Autodesk Fusion 360 part; units mm, degrees
(part 23 of 40)
  line L3449 (13.3622, 59.5542) -> (13.369, 59.5843) construction
  line L3450 (13.369, 59.5843) -> (13.3833, 59.6444) construction
  line L3451 (13.3833, 59.6444) -> (13.4071, 59.7338) construction
  line L3452 (13.4071, 59.7338) -> (13.4435, 59.8517) construction
  line L3453 (13.4435, 59.8517) -> (13.4951, 59.9973) construction
  line L3454 (13.4951, 59.9973) -> (13.5511, 60.1416) construction
  line L3455 (13.5511, 60.1416) -> (13.6099, 60.2852) construction
  line L3456 (13.6099, 60.2852) -> (13.6701, 60.4283) construction
  line L3457 (13.6701, 60.4283) -> (13.7313, 60.5711) construction
  line L3458 (13.7313, 60.5711) -> (13.7935, 60.7136) construction
  line L3459 (13.7935, 60.7136) -> (13.8571, 60.8557) construction
  line L3460 (13.8571, 60.8557) -> (13.9226, 60.9971) construction
  line L3461 (13.9226, 60.9971) -> (13.9902, 61.1379) construction
  line L3462 (13.9902, 61.1379) -> (14.06, 61.2779) construction
  line L3463 (14.06, 61.2779) -> (14.1316, 61.4173) construction
  line L3464 (14.1316, 61.4173) -> (14.205, 61.5561) construction
  line L3465 (14.205, 61.5561) -> (14.2797, 61.6944) construction
  line L3466 (14.2797, 61.6944) -> (14.3557, 61.8322) construction
  line L3467 (14.3557, 61.8322) -> (14.4327, 61.9697) construction
  line L3468 (14.4327, 61.9697) -> (14.5109, 62.1067) construction
  line L3469 (14.5109, 62.1067) -> (14.5904, 62.2432) construction
  line L3470 (14.5904, 62.2432) -> (14.6711, 62.3792) construction
  line L3471 (14.6711, 62.3792) -> (14.753, 62.5148) construction
  line L3472 (14.753, 62.5148) -> (14.8363, 62.6498) construction
  line L3473 (14.8363, 62.6498) -> (14.9208, 62.7843) construction
  line L3474 (14.9208, 62.7843) -> (15.0064, 62.9184) construction
  line L3475 (15.0064, 62.9184) -> (15.0932, 63.052) construction
  line L3476 (15.0932, 63.052) -> (15.181, 63.1852) construction
  line L3477 (15.181, 63.1852) -> (15.2698, 63.318) construction
  line L3478 (15.2698, 63.318) -> (15.3597, 63.4503) construction
  line L3479 (15.3597, 63.4503) -> (15.4506, 63.5821) construction
  line L3480 (15.4506, 63.5821) -> (15.5425, 63.7135) construction
  line L3481 (15.5425, 63.7135) -> (15.6354, 63.8445) construction
  line L3482 (15.6354, 63.8445) -> (15.7293, 63.975) construction
  line L3483 (15.7293, 63.975) -> (15.8242, 64.105) construction
  line L3484 (15.8242, 64.105) -> (15.92, 64.2346) construction
  line L3485 (15.92, 64.2346) -> (16.0168, 64.3638) construction
  line L3486 (16.0168, 64.3638) -> (16.1146, 64.4926) construction
  line L3487 (16.1146, 64.4926) -> (16.2132, 64.6209) construction
  line L3488 (16.2132, 64.6209) -> (16.3127, 64.7488) construction
  line L3489 (16.3127, 64.7488) -> (16.4131, 64.8762) construction
  line L3490 (16.4131, 64.8762) -> (16.5144, 65.0032) construction
  line L3491 (16.5144, 65.0032) -> (16.6166, 65.1298) construction
  line L3492 (16.6166, 65.1298) -> (16.7196, 65.256) construction
  line L3493 (16.7196, 65.256) -> (16.8235, 65.3817) construction
  line L3494 (16.8235, 65.3817) -> (16.9283, 65.507) construction
  line L3495 (16.9283, 65.507) -> (17.0338, 65.6318) construction
  line L3496 (17.0338, 65.6318) -> (17.1402, 65.7562) construction
  line L3497 (17.1402, 65.7562) -> (17.2474, 65.8802) construction
  line L3498 (17.2474, 65.8802) -> (17.3555, 66.0038) construction
  line L3499 (17.3555, 66.0038) -> (17.4643, 66.1269) construction
  line L3500 (17.4643, 66.1269) -> (17.5739, 66.2497) construction
  line L3501 (17.5739, 66.2497) -> (17.6842, 66.3719) construction
  line L3502 (17.6842, 66.3719) -> (17.7954, 66.4938) construction
  line L3503 (17.7954, 66.4938) -> (17.9073, 66.6152) construction
  line L3504 (17.9073, 66.6152) -> (18.02, 66.7362) construction
  line L3505 (18.02, 66.7362) -> (18.1335, 66.8568) construction
  line L3506 (18.1335, 66.8568) -> (18.2477, 66.9769) construction
  line L3507 (18.2477, 66.9769) -> (18.3626, 67.0966) construction
  line L3508 (18.3626, 67.0966) -> (18.4782, 67.2159) construction
  line L3509 (18.4782, 67.2159) -> (18.5946, 67.3347) construction
  line L3510 (18.5946, 67.3347) -> (18.7118, 67.4531) construction
  line L3511 (18.7118, 67.4531) -> (18.8296, 67.5711) construction
  line L3512 (18.8296, 67.5711) -> (18.9481, 67.6887) construction
  line L3513 (18.9481, 67.6887) -> (19.0674, 67.8058) construction
  line L3514 (19.0674, 67.8058) -> (19.1873, 67.9225) construction
  line L3515 (19.1873, 67.9225) -> (19.3079, 68.0388) construction
  line L3516 (19.3079, 68.0388) -> (19.4293, 68.1546) construction
  line L3517 (19.4293, 68.1546) -> (19.5512, 68.27) construction
  line L3518 (19.5512, 68.27) -> (19.6739, 68.385) construction
  line L3519 (19.6739, 68.385) -> (19.7726, 68.4767) construction
  line L3520 (19.7726, 68.4767) -> (19.8469, 68.5452) construction
  line L3521 (19.8469, 68.5452) -> (19.8966, 68.5908) construction
  line L3522 (19.8966, 68.5908) -> (19.9215, 68.6136) construction
  spline S47 degree 5 poles (-52.5103, -31.1115) (-52.5368, -31.1272) (-52.5895, -31.1594) (-52.6672, -31.2097) (-52.7681, -31.2807) (-52.8906, -31.3748) (-53.0106, -31.4727) (-53.1289, -31.5729) (-53.2464, -31.6744) (-53.3634, -31.7767) (-53.4797, -31.88) (-53.5951, -31.9844) (-53.7094, -32.0903) (-53.8224, -32.1981) (-53.934, -32.3077) (-54.0444, -32.419) (-54.1537, -32.5316) (-54.2622, -32.6455) (-54.3698, -32.7603) (-54.4767, -32.876) (-54.5828, -32.9927) (-54.6881, -33.1105) (-54.7926, -33.2292) (-54.8961, -33.3491) (-54.9988, -33.47) (-55.1007, -33.5919) (-55.2017, -33.7148) (-55.302, -33.8386) (-55.4015, -33.9633) (-55.5003, -34.0888) (-55.5984, -34.2151) (-55.6957, -34.3423) (-55.7923, -34.4703) (-55.8881, -34.5991) (-55.9832, -34.7288) (-56.0776, -34.8592) (-56.1712, -34.9905) (-56.2642, -35.1224) (-56.3564, -35.2552) (-56.448, -35.3886) (-56.5388, -35.5228) (-56.629, -35.6577) (-56.7185, -35.7933) (-56.8073, -35.9295) (-56.8955, -36.0665) (-56.9829, -36.2042) (-57.0697, -36.3425) (-57.1558, -36.4815) (-57.2413, -36.6211) (-57.3261, -36.7614) (-57.4102, -36.9023) (-57.4937, -37.0438) (-57.5765, -37.186) (-57.6587, -37.3288) (-57.7403, -37.4721) (-57.8212, -37.6161) (-57.9014, -37.7607) (-57.981, -37.9058) (-58.06, -38.0515) (-58.1383, -38.1978) (-58.216, -38.3447) (-58.2931, -38.4921) (-58.3695, -38.6401) (-58.4453, -38.7886) (-58.5205, -38.9377) (-58.595, -39.0873) (-58.669, -39.2374) (-58.7423, -39.3881) (-58.8149, -39.5393) (-58.887, -39.6909) (-58.9584, -39.8431) (-59.0151, -39.9653) (-59.0573, -40.0572) (-59.0853, -40.1185) (-59.0993, -40.1492) knots 0 0 0 0 0 0 0.01428571 0.02857143 0.04285714 0.05714286 0.07142857 0.08571429 0.1 0.11428571 0.12857143 0.14285714 0.15714286 0.17142857 0.18571429 0.2 0.21428571 0.22857143 0.24285714 0.25714286 0.27142857 0.28571429 0.3 0.31428571 0.32857143 0.34285714 0.35714286 0.37142857 0.38571429 0.4 0.41428571 0.42857143 0.44285714 0.45714286 0.47142857 0.48571429 0.5 0.51428571 0.52857143 0.54285714 0.55714286 0.57142857 0.58571429 0.6 0.61428571 0.62857143 0.64285714 0.65714286 0.67142857 0.68571429 0.7 0.71428571 0.72857143 0.74285714 0.75714286 0.77142857 0.78571429 0.8 0.81428571 0.82857143 0.84285714 0.85714286 0.87142857 0.88571429 0.9 0.91428571 0.92857143 0.94285714 0.95714286 0.97142857 0.98571429 1 1 1 1 1 1
  line L3523 (-52.5103, -31.1115) -> (-52.5368, -31.1272) construction
  line L3524 (-52.5368, -31.1272) -> (-52.5895, -31.1594) construction
  line L3525 (-52.5895, -31.1594) -> (-52.6672, -31.2097) construction
  line L3526 (-52.6672, -31.2097) -> (-52.7681, -31.2807) construction
  line L3527 (-52.7681, -31.2807) -> (-52.8906, -31.3748) construction
  line L3528 (-52.8906, -31.3748) -> (-53.0106, -31.4727) construction
  line L3529 (-53.0106, -31.4727) -> (-53.1289, -31.5729) construction
  line L3530 (-53.1289, -31.5729) -> (-53.2464, -31.6744) construction
  line L3531 (-53.2464, -31.6744) -> (-53.3634, -31.7767) construction
  line L3532 (-53.3634, -31.7767) -> (-53.4797, -31.88) construction
  line L3533 (-53.4797, -31.88) -> (-53.5951, -31.9844) construction
  line L3534 (-53.5951, -31.9844) -> (-53.7094, -32.0903) construction
  line L3535 (-53.7094, -32.0903) -> (-53.8224, -32.1981) construction
  line L3536 (-53.8224, -32.1981) -> (-53.934, -32.3077) construction
  line L3537 (-53.934, -32.3077) -> (-54.0444, -32.419) construction
  line L3538 (-54.0444, -32.419) -> (-54.1537, -32.5316) construction
  line L3539 (-54.1537, -32.5316) -> (-54.2622, -32.6455) construction
  line L3540 (-54.2622, -32.6455) -> (-54.3698, -32.7603) construction
  line L3541 (-54.3698, -32.7603) -> (-54.4767, -32.876) construction
  line L3542 (-54.4767, -32.876) -> (-54.5828, -32.9927) construction
  line L3543 (-54.5828, -32.9927) -> (-54.6881, -33.1105) construction
  line L3544 (-54.6881, -33.1105) -> (-54.7926, -33.2292) construction
  line L3545 (-54.7926, -33.2292) -> (-54.8961, -33.3491) construction
  line L3546 (-54.8961, -33.3491) -> (-54.9988, -33.47) construction
  line L3547 (-54.9988, -33.47) -> (-55.1007, -33.5919) construction
  line L3548 (-55.1007, -33.5919) -> (-55.2017, -33.7148) construction
  line L3549 (-55.2017, -33.7148) -> (-55.302, -33.8386) construction
  line L3550 (-55.302, -33.8386) -> (-55.4015, -33.9633) construction
  line L3551 (-55.4015, -33.9633) -> (-55.5003, -34.0888) construction
  line L3552 (-55.5003, -34.0888) -> (-55.5984, -34.2151) construction
  line L3553 (-55.5984, -34.2151) -> (-55.6957, -34.3423) construction
  line L3554 (-55.6957, -34.3423) -> (-55.7923, -34.4703) construction
  line L3555 (-55.7923, -34.4703) -> (-55.8881, -34.5991) construction
  line L3556 (-55.8881, -34.5991) -> (-55.9832, -34.7288) construction
  line L3557 (-55.9832, -34.7288) -> (-56.0776, -34.8592) construction
  line L3558 (-56.0776, -34.8592) -> (-56.1712, -34.9905) construction
  line L3559 (-56.1712, -34.9905) -> (-56.2642, -35.1224) construction
  line L3560 (-56.2642, -35.1224) -> (-56.3564, -35.2552) construction
  line L3561 (-56.3564, -35.2552) -> (-56.448, -35.3886) construction
  line L3562 (-56.448, -35.3886) -> (-56.5388, -35.5228) construction
  line L3563 (-56.5388, -35.5228) -> (-56.629, -35.6577) construction
  line L3564 (-56.629, -35.6577) -> (-56.7185, -35.7933) construction
  line L3565 (-56.7185, -35.7933) -> (-56.8073, -35.9295) construction
  line L3566 (-56.8073, -35.9295) -> (-56.8955, -36.0665) construction
  line L3567 (-56.8955, -36.0665) -> (-56.9829, -36.2042) construction
  line L3568 (-56.9829, -36.2042) -> (-57.0697, -36.3425) construction
  line L3569 (-57.0697, -36.3425) -> (-57.1558, -36.4815) construction
  line L3570 (-57.1558, -36.4815) -> (-57.2413, -36.6211) construction
  line L3571 (-57.2413, -36.6211) -> (-57.3261, -36.7614) construction
  line L3572 (-57.3261, -36.7614) -> (-57.4102, -36.9023) construction
  line L3573 (-57.4102, -36.9023) -> (-57.4937, -37.0438) construction
  line L3574 (-57.4937, -37.0438) -> (-57.5765, -37.186) construction
  line L3575 (-57.5765, -37.186) -> (-57.6587, -37.3288) construction
  line L3576 (-57.6587, -37.3288) -> (-57.7403, -37.4721) construction
  line L3577 (-57.7403, -37.4721) -> (-57.8212, -37.6161) construction
  line L3578 (-57.8212, -37.6161) -> (-57.9014, -37.7607) construction
  line L3579 (-57.9014, -37.7607) -> (-57.981, -37.9058) construction
  line L3580 (-57.981, -37.9058) -> (-58.06, -38.0515) construction
  line L3581 (-58.06, -38.0515) -> (-58.1383, -38.1978) construction
  line L3582 (-58.1383, -38.1978) -> (-58.216, -38.3447) construction
  line L3583 (-58.216, -38.3447) -> (-58.2931, -38.4921) construction
  line L3584 (-58.2931, -38.4921) -> (-58.3695, -38.6401) construction
  line L3585 (-58.3695, -38.6401) -> (-58.4453, -38.7886) construction
  line L3586 (-58.4453, -38.7886) -> (-58.5205, -38.9377) construction
  line L3587 (-58.5205, -38.9377) -> (-58.595, -39.0873) construction
  line L3588 (-58.595, -39.0873) -> (-58.669, -39.2374) construction
  line L3589 (-58.669, -39.2374) -> (-58.7423, -39.3881) construction
  line L3590 (-58.7423, -39.3881) -> (-58.8149, -39.5393) construction
  line L3591 (-58.8149, -39.5393) -> (-58.887, -39.6909) construction
  line L3592 (-58.887, -39.6909) -> (-58.9584, -39.8431) construction
  line L3593 (-58.9584, -39.8431) -> (-59.0151, -39.9653) construction
  line L3594 (-59.0151, -39.9653) -> (-59.0573, -40.0572) construction
  line L3595 (-59.0573, -40.0572) -> (-59.0853, -40.1185) construction
  line L3596 (-59.0853, -40.1185) -> (-59.0993, -40.1492) construction
  arc A87 (-39.2483, -44.5906) -> (-39.3784, -41.8132) centre (-40.7496, -43.2692) ccw
  arc A88 (10.6816, 56.435) -> (13.005, 57.9623) centre (11.0535, 58.4001) ccw
  arc A89 (68.6136, 19.9215) -> (67.2191, 24.2132) centre (0, 0) ccw
  arc A90 (27.5982, 50.3721) -> (30.2798, 51.1066) centre (28.5592, 52.1261) ccw
  spline S48 degree 5 poles (60.7685, -5.6951) (60.7993, -5.6979) (60.8609, -5.7029) (60.9533, -5.7078) (61.0766, -5.7097) (61.231, -5.7056) (61.3856, -5.6969) (61.5403, -5.6854) (61.695, -5.6723) (61.8498, -5.6583) (62.0045, -5.6431) (62.1593, -5.6265) (62.314, -5.608) (62.4688, -5.5871) (62.6235, -5.5641) (62.7782, -5.539) (62.9329, -5.5121) (63.0875, -5.4838) (63.2421, -5.4542) (63.3966, -5.4233) (63.5511, -5.3913) (63.7055, -5.3579) (63.8598, -5.3232) (64.014, -5.2871) (64.1682, -5.2497) (64.3222, -5.2109) (64.4762, -5.1709) (64.6301, -5.1297) (64.7839, -5.0873) (64.9376, -5.0439) (65.0912, -4.9993) (65.2447, -4.9536) (65.398, -4.9068) (65.5513, -4.8589) (65.7044, -4.8099) (65.8574, -4.7599) (66.0103, -4.7087) (66.1631, -4.6566) (66.3158, -4.6035) (66.4683, -4.5493) (66.6206, -4.4942) (66.7729, -4.438) (66.925, -4.381) (67.077, -4.3229) (67.2288, -4.2639) (67.3804, -4.2039) (67.532, -4.143) (67.6833, -4.0812) (67.8345, -4.0185) (67.9856, -3.9548) (68.1365, -3.8903) (68.2872, -3.8249) (68.4378, -3.7585) (68.5882, -3.6913) (68.7384, -3.6233) (68.8885, -3.5543) (69.0384, -3.4846) (69.1881, -3.4139) (69.3376, -3.3425) (69.487, -3.2701) (69.6362, -3.197) (69.7852, -3.123) (69.934, -3.0482) (70.0826, -2.9726) (70.2311, -2.8962) (70.3793, -2.819) (70.5274, -2.741) (70.6752, -2.6622) (70.8229, -2.5826) (70.9703, -2.5023) (71.1176, -2.4211) (71.2352, -2.3556) (71.3234, -2.3061) (71.3821, -2.2729) (71.4115, -2.2563) knots 0 0 0 0 0 0 0.01428571 0.02857143 0.04285714 0.05714286 0.07142857 0.08571429 0.1 0.11428571 0.12857143 0.14285714 0.15714286 0.17142857 0.18571429 0.2 0.21428571 0.22857143 0.24285714 0.25714286 0.27142857 0.28571429 0.3 0.31428571 0.32857143 0.34285714 0.35714286 0.37142857 0.38571429 0.4 0.41428571 0.42857143 0.44285714 0.45714286 0.47142857 0.48571429 0.5 0.51428571 0.52857143 0.54285714 0.55714286 0.57142857 0.58571429 0.6 0.61428571 0.62857143 0.64285714 0.65714286 0.67142857 0.68571429 0.7 0.71428571 0.72857143 0.74285714 0.75714286 0.77142857 0.78571429 0.8 0.81428571 0.82857143 0.84285714 0.85714286 0.87142857 0.88571429 0.9 0.91428571 0.92857143 0.94285714 0.95714286 0.97142857 0.98571429 1 1 1 1 1 1
  line L3597 (60.7685, -5.6951) -> (60.7993, -5.6979) construction
  line L3598 (60.7993, -5.6979) -> (60.8609, -5.7029) construction
  line L3599 (60.8609, -5.7029) -> (60.9533, -5.7078) construction
  line L3600 (60.9533, -5.7078) -> (61.0766, -5.7097) construction
  line L3601 (61.0766, -5.7097) -> (61.231, -5.7056) construction
  line L3602 (61.231, -5.7056) -> (61.3856, -5.6969) construction
  line L3603 (61.3856, -5.6969) -> (61.5403, -5.6854) construction
  line L3604 (61.5403, -5.6854) -> (61.695, -5.6723) construction
  line L3605 (61.695, -5.6723) -> (61.8498, -5.6583) construction
  line L3606 (61.8498, -5.6583) -> (62.0045, -5.6431) construction
  line L3607 (62.0045, -5.6431) -> (62.1593, -5.6265) construction
  line L3608 (62.1593, -5.6265) -> (62.314, -5.608) construction
  line L3609 (62.314, -5.608) -> (62.4688, -5.5871) construction
  line L3610 (62.4688, -5.5871) -> (62.6235, -5.5641) construction
  line L3611 (62.6235, -5.5641) -> (62.7782, -5.539) construction
  line L3612 (62.7782, -5.539) -> (62.9329, -5.5121) construction
  line L3613 (62.9329, -5.5121) -> (63.0875, -5.4838) construction
  line L3614 (63.0875, -5.4838) -> (63.2421, -5.4542) construction
  line L3615 (63.2421, -5.4542) -> (63.3966, -5.4233) construction
  line L3616 (63.3966, -5.4233) -> (63.5511, -5.3913) construction
  line L3617 (63.5511, -5.3913) -> (63.7055, -5.3579) construction
  line L3618 (63.7055, -5.3579) -> (63.8598, -5.3232) construction
  line L3619 (63.8598, -5.3232) -> (64.014, -5.2871) construction
  line L3620 (64.014, -5.2871) -> (64.1682, -5.2497) construction
  line L3621 (64.1682, -5.2497) -> (64.3222, -5.2109) construction
  line L3622 (64.3222, -5.2109) -> (64.4762, -5.1709) construction
  line L3623 (64.4762, -5.1709) -> (64.6301, -5.1297) construction
  line L3624 (64.6301, -5.1297) -> (64.7839, -5.0873) construction
  line L3625 (64.7839, -5.0873) -> (64.9376, -5.0439) construction
  line L3626 (64.9376, -5.0439) -> (65.0912, -4.9993) construction
  line L3627 (65.0912, -4.9993) -> (65.2447, -4.9536) construction
  line L3628 (65.2447, -4.9536) -> (65.398, -4.9068) construction
  line L3629 (65.398, -4.9068) -> (65.5513, -4.8589) construction
  line L3630 (65.5513, -4.8589) -> (65.7044, -4.8099) construction
  line L3631 (65.7044, -4.8099) -> (65.8574, -4.7599) construction
  line L3632 (65.8574, -4.7599) -> (66.0103, -4.7087) construction
  line L3633 (66.0103, -4.7087) -> (66.1631, -4.6566) construction
  line L3634 (66.1631, -4.6566) -> (66.3158, -4.6035) construction
  line L3635 (66.3158, -4.6035) -> (66.4683, -4.5493) construction
  line L3636 (66.4683, -4.5493) -> (66.6206, -4.4942) construction
  line L3637 (66.6206, -4.4942) -> (66.7729, -4.438) construction
  line L3638 (66.7729, -4.438) -> (66.925, -4.381) construction
  line L3639 (66.925, -4.381) -> (67.077, -4.3229) construction
  line L3640 (67.077, -4.3229) -> (67.2288, -4.2639) construction
  line L3641 (67.2288, -4.2639) -> (67.3804, -4.2039) construction
  line L3642 (67.3804, -4.2039) -> (67.532, -4.143) construction
  line L3643 (67.532, -4.143) -> (67.6833, -4.0812) construction
  line L3644 (67.6833, -4.0812) -> (67.8345, -4.0185) construction
  line L3645 (67.8345, -4.0185) -> (67.9856, -3.9548) construction
  line L3646 (67.9856, -3.9548) -> (68.1365, -3.8903) construction
  line L3647 (68.1365, -3.8903) -> (68.2872, -3.8249) construction
  line L3648 (68.2872, -3.8249) -> (68.4378, -3.7585) construction
  line L3649 (68.4378, -3.7585) -> (68.5882, -3.6913) construction
  line L3650 (68.5882, -3.6913) -> (68.7384, -3.6233) construction
  line L3651 (68.7384, -3.6233) -> (68.8885, -3.5543) construction
  line L3652 (68.8885, -3.5543) -> (69.0384, -3.4846) construction
  line L3653 (69.0384, -3.4846) -> (69.1881, -3.4139) construction
  line L3654 (69.1881, -3.4139) -> (69.3376, -3.3425) construction
  line L3655 (69.3376, -3.3425) -> (69.487, -3.2701) construction
  line L3656 (69.487, -3.2701) -> (69.6362, -3.197) construction
  line L3657 (69.6362, -3.197) -> (69.7852, -3.123) construction
  line L3658 (69.7852, -3.123) -> (69.934, -3.0482) construction
  line L3659 (69.934, -3.0482) -> (70.0826, -2.9726) construction
  line L3660 (70.0826, -2.9726) -> (70.2311, -2.8962) construction
  line L3661 (70.2311, -2.8962) -> (70.3793, -2.819) construction
  line L3662 (70.3793, -2.819) -> (70.5274, -2.741) construction
  line L3663 (70.5274, -2.741) -> (70.6752, -2.6622) construction
  line L3664 (70.6752, -2.6622) -> (70.8229, -2.5826) construction
  line L3665 (70.8229, -2.5826) -> (70.9703, -2.5023) construction
  line L3666 (70.9703, -2.5023) -> (71.1176, -2.4211) construction
  line L3667 (71.1176, -2.4211) -> (71.2352, -2.3556) construction
  line L3668 (71.2352, -2.3556) -> (71.3234, -2.3061) construction
  line L3669 (71.3234, -2.3061) -> (71.3821, -2.2729) construction
  line L3670 (71.3821, -2.2729) -> (71.4115, -2.2563) construction
  spline S49 degree 5 poles (40.3263, -45.8153) (40.3467, -45.8385) (40.3868, -45.8854) (40.4451, -45.9573) (40.5192, -46.056) (40.6066, -46.1833) (40.6904, -46.3135) (40.772, -46.4454) (40.8524, -46.5782) (40.932, -46.7117) (41.0107, -46.8458) (41.0883, -46.9807) (41.1642, -47.1168) (41.2383, -47.2543) (41.3106, -47.393) (41.3813, -47.5329) (41.4504, -47.6738) (41.5184, -47.8156) (41.5853, -47.9581) (41.6512, -48.1012) (41.716, -48.245) (41.7798, -48.3895) (41.8424, -48.5347) (41.9039, -48.6807) (41.9642, -48.8274) (42.0234, -48.9749) (42.0815, -49.123) (42.1386, -49.2717) (42.1947, -49.421) (42.2499, -49.5709) (42.3041, -49.7214) (42.3574, -49.8724) (42.4097, -50.024) (42.461, -50.1761) (42.5114, -50.3288) (42.5608, -50.482) (42.6094, -50.6358) (42.657, -50.79) (42.7037, -50.9447) (42.7495, -51.0999) (42.7945, -51.2556) (42.8386, -51.4118) (42.8818, -51.5684) (42.9241, -51.7255) (42.9656, -51.883) (43.0063, -52.0409) (43.0461, -52.1993) (43.085, -52.3581) (43.1231, -52.5173) (43.1604, -52.6769) (43.1969, -52.8369) (43.2326, -52.9973) (43.2674, -53.1581) (43.3015, -53.3193) (43.3347, -53.4809) (43.3672, -53.6428) (43.3988, -53.8051) (43.4297, -53.9677) (43.4597, -54.1307) (43.489, -54.294) (43.5175, -54.4577) (43.5453, -54.6217) (43.5723, -54.7861) (43.5984, -54.9508) (43.6239, -55.1158) (43.6486, -55.2811) (43.6725, -55.4467) (43.6956, -55.6126) (43.718, -55.7789) (43.7397, -55.9454) (43.7606, -56.1122) (43.7767, -56.2459) (43.7885, -56.3463) (43.7962, -56.4133) (43.8, -56.4469) knots 0 0 0 0 0 0 0.01428571 0.02857143 0.04285714 0.05714286 0.07142857 0.08571429 0.1 0.11428571 0.12857143 0.14285714 0.15714286 0.17142857 0.18571429 0.2 0.21428571 0.22857143 0.24285714 0.25714286 0.27142857 0.28571429 0.3 0.31428571 0.32857143 0.34285714 0.35714286 0.37142857 0.38571429 0.4 0.41428571 0.42857143 0.44285714 0.45714286 0.47142857 0.48571429 0.5 0.51428571 0.52857143 0.54285714 0.55714286 0.57142857 0.58571429 0.6 0.61428571 0.62857143 0.64285714 0.65714286 0.67142857 0.68571429 0.7 0.71428571 0.72857143 0.74285714 0.75714286 0.77142857 0.78571429 0.8 0.81428571 0.82857143 0.84285714 0.85714286 0.87142857 0.88571429 0.9 0.91428571 0.92857143 0.94285714 0.95714286 0.97142857 0.98571429 1 1 1 1 1 1
  line L3671 (40.3263, -45.8153) -> (40.3467, -45.8385) construction
  line L3672 (40.3467, -45.8385) -> (40.3868, -45.8854) construction
  line L3673 (40.3868, -45.8854) -> (40.4451, -45.9573) construction
  line L3674 (40.4451, -45.9573) -> (40.5192, -46.056) construction
  line L3675 (40.5192, -46.056) -> (40.6066, -46.1833) construction
  line L3676 (40.6066, -46.1833) -> (40.6904, -46.3135) construction
  line L3677 (40.6904, -46.3135) -> (40.772, -46.4454) construction
  line L3678 (40.772, -46.4454) -> (40.8524, -46.5782) construction
  line L3679 (40.8524, -46.5782) -> (40.932, -46.7117) construction
  line L3680 (40.932, -46.7117) -> (41.0107, -46.8458) construction
  line L3681 (41.0107, -46.8458) -> (41.0883, -46.9807) construction
  line L3682 (41.0883, -46.9807) -> (41.1642, -47.1168) construction
  line L3683 (41.1642, -47.1168) -> (41.2383, -47.2543) construction
  line L3684 (41.2383, -47.2543) -> (41.3106, -47.393) construction
  line L3685 (41.3106, -47.393) -> (41.3813, -47.5329) construction
  line L3686 (41.3813, -47.5329) -> (41.4504, -47.6738) construction
  line L3687 (41.4504, -47.6738) -> (41.5184, -47.8156) construction
  line L3688 (41.5184, -47.8156) -> (41.5853, -47.9581) construction
  line L3689 (41.5853, -47.9581) -> (41.6512, -48.1012) construction
  line L3690 (41.6512, -48.1012) -> (41.716, -48.245) construction
  line L3691 (41.716, -48.245) -> (41.7798, -48.3895) construction
  line L3692 (41.7798, -48.3895) -> (41.8424, -48.5347) construction
  line L3693 (41.8424, -48.5347) -> (41.9039, -48.6807) construction
  line L3694 (41.9039, -48.6807) -> (41.9642, -48.8274) construction
  line L3695 (41.9642, -48.8274) -> (42.0234, -48.9749) construction
  line L3696 (42.0234, -48.9749) -> (42.0815, -49.123) construction
  line L3697 (42.0815, -49.123) -> (42.1386, -49.2717) construction
  line L3698 (42.1386, -49.2717) -> (42.1947, -49.421) construction
  line L3699 (42.1947, -49.421) -> (42.2499, -49.5709) construction
  line L3700 (42.2499, -49.5709) -> (42.3041, -49.7214) construction
  line L3701 (42.3041, -49.7214) -> (42.3574, -49.8724) construction
  line L3702 (42.3574, -49.8724) -> (42.4097, -50.024) construction
  line L3703 (42.4097, -50.024) -> (42.461, -50.1761) construction
  line L3704 (42.461, -50.1761) -> (42.5114, -50.3288) construction
  line L3705 (42.5114, -50.3288) -> (42.5608, -50.482) construction
  line L3706 (42.5608, -50.482) -> (42.6094, -50.6358) construction
  line L3707 (42.6094, -50.6358) -> (42.657, -50.79) construction
  line L3708 (42.657, -50.79) -> (42.7037, -50.9447) construction
  line L3709 (42.7037, -50.9447) -> (42.7495, -51.0999) construction
  line L3710 (42.7495, -51.0999) -> (42.7945, -51.2556) construction
  line L3711 (42.7945, -51.2556) -> (42.8386, -51.4118) construction
  line L3712 (42.8386, -51.4118) -> (42.8818, -51.5684) construction
  line L3713 (42.8818, -51.5684) -> (42.9241, -51.7255) construction
  line L3714 (42.9241, -51.7255) -> (42.9656, -51.883) construction
  line L3715 (42.9656, -51.883) -> (43.0063, -52.0409) construction
  line L3716 (43.0063, -52.0409) -> (43.0461, -52.1993) construction
  line L3717 (43.0461, -52.1993) -> (43.085, -52.3581) construction
  line L3718 (43.085, -52.3581) -> (43.1231, -52.5173) construction
  line L3719 (43.1231, -52.5173) -> (43.1604, -52.6769) construction
  line L3720 (43.1604, -52.6769) -> (43.1969, -52.8369) construction
  line L3721 (43.1969, -52.8369) -> (43.2326, -52.9973) construction
  line L3722 (43.2326, -52.9973) -> (43.2674, -53.1581) construction
  line L3723 (43.2674, -53.1581) -> (43.3015, -53.3193) construction
  line L3724 (43.3015, -53.3193) -> (43.3347, -53.4809) construction
  line L3725 (43.3347, -53.4809) -> (43.3672, -53.6428) construction
  line L3726 (43.3672, -53.6428) -> (43.3988, -53.8051) construction
  line L3727 (43.3988, -53.8051) -> (43.4297, -53.9677) construction
  line L3728 (43.4297, -53.9677) -> (43.4597, -54.1307) construction
  line L3729 (43.4597, -54.1307) -> (43.489, -54.294) construction
  line L3730 (43.489, -54.294) -> (43.5175, -54.4577) construction
  line L3731 (43.5175, -54.4577) -> (43.5453, -54.6217) construction
  line L3732 (43.5453, -54.6217) -> (43.5723, -54.7861) construction
  line L3733 (43.5723, -54.7861) -> (43.5984, -54.9508) construction
  line L3734 (43.5984, -54.9508) -> (43.6239, -55.1158) construction
  line L3735 (43.6239, -55.1158) -> (43.6486, -55.2811) construction
  line L3736 (43.6486, -55.2811) -> (43.6725, -55.4467) construction
  line L3737 (43.6725, -55.4467) -> (43.6956, -55.6126) construction
  line L3738 (43.6956, -55.6126) -> (43.718, -55.7789) construction
  line L3739 (43.718, -55.7789) -> (43.7397, -55.9454) construction
  line L3740 (43.7397, -55.9454) -> (43.7606, -56.1122) construction
  line L3741 (43.7606, -56.1122) -> (43.7767, -56.2459) construction
  line L3742 (43.7767, -56.2459) -> (43.7885, -56.3463) construction
  line L3743 (43.7885, -56.3463) -> (43.7962, -56.4133) construction
  line L3744 (43.7962, -56.4133) -> (43.8, -56.4469) construction
  line L3745 (-5.5428, 59.1442) -> (-5.6951, 60.7685)
  arc A91 (51.9354, 24.5301) -> (50.3721, 27.5982) centre (0, 0) ccw
  arc A92 (24.5301, -51.9354) -> (23.5481, -54.5366) centre (25.3842, -53.7438) ccw
  spline S50 degree 5 poles (-13.3622, -59.5542) (-13.369, -59.5843) (-13.3833, -59.6444) (-13.4071, -59.7338) (-13.4435, -59.8517) (-13.4951, -59.9973) (-13.5511, -60.1416) (-13.6099, -60.2852) (-13.6701, -60.4283) (-13.7313, -60.5711) (-13.7935, -60.7136) (-13.8571, -60.8557) (-13.9226, -60.9971) (-13.9902, -61.1379) (-14.06, -61.2779) (-14.1316, -61.4173) (-14.205, -61.5561) (-14.2797, -61.6944) (-14.3557, -61.8322) (-14.4327, -61.9697) (-14.5109, -62.1067) (-14.5904, -62.2432) (-14.6711, -62.3792) (-14.753, -62.5148) (-14.8363, -62.6498) (-14.9208, -62.7843) (-15.0064, -62.9184) (-15.0932, -63.052) (-15.181, -63.1852) (-15.2698, -63.318) (-15.3597, -63.4503) (-15.4506, -63.5821) (-15.5425, -63.7135) (-15.6354, -63.8445) (-15.7293, -63.975) (-15.8242, -64.105) (-15.92, -64.2346) (-16.0168, -64.3638) (-16.1146, -64.4926) (-16.2132, -64.6209) (-16.3127, -64.7488) (-16.4131, -64.8762) (-16.5144, -65.0032) (-16.6166, -65.1298) (-16.7196, -65.256) (-16.8235, -65.3817) (-16.9283, -65.507) (-17.0338, -65.6318) (-17.1402, -65.7562) (-17.2474, -65.8802) (-17.3555, -66.0038) (-17.4643, -66.1269) (-17.5739, -66.2497) (-17.6842, -66.3719) (-17.7954, -66.4938) (-17.9073, -66.6152) (-18.02, -66.7362) (-18.1335, -66.8568) (-18.2477, -66.9769) (-18.3626, -67.0966) (-18.4782, -67.2159) (-18.5946, -67.3347) (-18.7118, -67.4531) (-18.8296, -67.5711) (-18.9481, -67.6887) (-19.0674, -67.8058) (-19.1873, -67.9225) (-19.3079, -68.0388) (-19.4293, -68.1546) (-19.5512, -68.27) (-19.6739, -68.385) (-19.7726, -68.4767) (-19.8469, -68.5452) (-19.8966, -68.5908) (-19.9215, -68.6136) knots 0 0 0 0 0 0 0.01428571 0.02857143 0.04285714 0.05714286 0.07142857 0.08571429 0.1 0.11428571 0.12857143 0.14285714 0.15714286 0.17142857 0.18571429 0.2 0.21428571 0.22857143 0.24285714 0.25714286 0.27142857 0.28571429 0.3 0.31428571 0.32857143 0.34285714 0.35714286 0.37142857 0.38571429 0.4 0.41428571 0.42857143 0.44285714 0.45714286 0.47142857 0.48571429 0.5 0.51428571 0.52857143 0.54285714 0.55714286 0.57142857 0.58571429 0.6 0.61428571 0.62857143 0.64285714 0.65714286 0.67142857 0.68571429 0.7 0.71428571 0.72857143 0.74285714 0.75714286 0.77142857 0.78571429 0.8 0.81428571 0.82857143 0.84285714 0.85714286 0.87142857 0.88571429 0.9 0.91428571 0.92857143 0.94285714 0.95714286 0.97142857 0.98571429 1 1 1 1 1 1
  line L3746 (-13.3622, -59.5542) -> (-13.369, -59.5843) construction
  line L3747 (-13.369, -59.5843) -> (-13.3833, -59.6444) construction
  line L3748 (-13.3833, -59.6444) -> (-13.4071, -59.7338) construction
  line L3749 (-13.4071, -59.7338) -> (-13.4435, -59.8517) construction
  line L3750 (-13.4435, -59.8517) -> (-13.4951, -59.9973) construction
  line L3751 (-13.4951, -59.9973) -> (-13.5511, -60.1416) construction
  line L3752 (-13.5511, -60.1416) -> (-13.6099, -60.2852) construction
  line L3753 (-13.6099, -60.2852) -> (-13.6701, -60.4283) construction
  line L3754 (-13.6701, -60.4283) -> (-13.7313, -60.5711) construction
  line L3755 (-13.7313, -60.5711) -> (-13.7935, -60.7136) construction
  line L3756 (-13.7935, -60.7136) -> (-13.8571, -60.8557) construction
  line L3757 (-13.8571, -60.8557) -> (-13.9226, -60.9971) construction
  line L3758 (-13.9226, -60.9971) -> (-13.9902, -61.1379) construction
  line L3759 (-13.9902, -61.1379) -> (-14.06, -61.2779) construction
  line L3760 (-14.06, -61.2779) -> (-14.1316, -61.4173) construction
  line L3761 (-14.1316, -61.4173) -> (-14.205, -61.5561) construction
  line L3762 (-14.205, -61.5561) -> (-14.2797, -61.6944) construction
  line L3763 (-14.2797, -61.6944) -> (-14.3557, -61.8322) construction
  line L3764 (-14.3557, -61.8322) -> (-14.4327, -61.9697) construction
  line L3765 (-14.4327, -61.9697) -> (-14.5109, -62.1067) construction
  line L3766 (-14.5109, -62.1067) -> (-14.5904, -62.2432) construction
  line L3767 (-14.5904, -62.2432) -> (-14.6711, -62.3792) construction
  line L3768 (-14.6711, -62.3792) -> (-14.753, -62.5148) construction
  line L3769 (-14.753, -62.5148) -> (-14.8363, -62.6498) construction
  line L3770 (-14.8363, -62.6498) -> (-14.9208, -62.7843) construction
  line L3771 (-14.9208, -62.7843) -> (-15.0064, -62.9184) construction
  line L3772 (-15.0064, -62.9184) -> (-15.0932, -63.052) construction
  line L3773 (-15.0932, -63.052) -> (-15.181, -63.1852) construction
  line L3774 (-15.181, -63.1852) -> (-15.2698, -63.318) construction
  line L3775 (-15.2698, -63.318) -> (-15.3597, -63.4503) construction
  line L3776 (-15.3597, -63.4503) -> (-15.4506, -63.5821) construction
  line L3777 (-15.4506, -63.5821) -> (-15.5425, -63.7135) construction
  line L3778 (-15.5425, -63.7135) -> (-15.6354, -63.8445) construction
  line L3779 (-15.6354, -63.8445) -> (-15.7293, -63.975) construction
  line L3780 (-15.7293, -63.975) -> (-15.8242, -64.105) construction
  line L3781 (-15.8242, -64.105) -> (-15.92, -64.2346) construction
  line L3782 (-15.92, -64.2346) -> (-16.0168, -64.3638) construction
  line L3783 (-16.0168, -64.3638) -> (-16.1146, -64.4926) construction
  line L3784 (-16.1146, -64.4926) -> (-16.2132, -64.6209) construction
  line L3785 (-16.2132, -64.6209) -> (-16.3127, -64.7488) construction
  line L3786 (-16.3127, -64.7488) -> (-16.4131, -64.8762) construction
  line L3787 (-16.4131, -64.8762) -> (-16.5144, -65.0032) construction
  line L3788 (-16.5144, -65.0032) -> (-16.6166, -65.1298) construction
  line L3789 (-16.6166, -65.1298) -> (-16.7196, -65.256) construction
  line L3790 (-16.7196, -65.256) -> (-16.8235, -65.3817) construction
  line L3791 (-16.8235, -65.3817) -> (-16.9283, -65.507) construction
  line L3792 (-16.9283, -65.507) -> (-17.0338, -65.6318) construction
  line L3793 (-17.0338, -65.6318) -> (-17.1402, -65.7562) construction
  line L3794 (-17.1402, -65.7562) -> (-17.2474, -65.8802) construction
  line L3795 (-17.2474, -65.8802) -> (-17.3555, -66.0038) construction
  line L3796 (-17.3555, -66.0038) -> (-17.4643, -66.1269) construction
  line L3797 (-17.4643, -66.1269) -> (-17.5739, -66.2497) construction
  line L3798 (-17.5739, -66.2497) -> (-17.6842, -66.3719) construction
  line L3799 (-17.6842, -66.3719) -> (-17.7954, -66.4938) construction
  line L3800 (-17.7954, -66.4938) -> (-17.9073, -66.6152) construction
  line L3801 (-17.9073, -66.6152) -> (-18.02, -66.7362) construction
  line L3802 (-18.02, -66.7362) -> (-18.1335, -66.8568) construction
  line L3803 (-18.1335, -66.8568) -> (-18.2477, -66.9769) construction
  line L3804 (-18.2477, -66.9769) -> (-18.3626, -67.0966) construction
  line L3805 (-18.3626, -67.0966) -> (-18.4782, -67.2159) construction
  line L3806 (-18.4782, -67.2159) -> (-18.5946, -67.3347) construction
  line L3807 (-18.5946, -67.3347) -> (-18.7118, -67.4531) construction
  line L3808 (-18.7118, -67.4531) -> (-18.8296, -67.5711) construction
  line L3809 (-18.8296, -67.5711) -> (-18.9481, -67.6887) construction
  line L3810 (-18.9481, -67.6887) -> (-19.0674, -67.8058) construction
  line L3811 (-19.0674, -67.8058) -> (-19.1873, -67.9225) construction
  line L3812 (-19.1873, -67.9225) -> (-19.3079, -68.0388) construction
  line L3813 (-19.3079, -68.0388) -> (-19.4293, -68.1546) construction
  line L3814 (-19.4293, -68.1546) -> (-19.5512, -68.27) construction
  line L3815 (-19.5512, -68.27) -> (-19.6739, -68.385) construction
  line L3816 (-19.6739, -68.385) -> (-19.7726, -68.4767) construction
  line L3817 (-19.7726, -68.4767) -> (-19.8469, -68.5452) construction
  line L3818 (-19.8469, -68.5452) -> (-19.8966, -68.5908) construction
  line L3819 (-19.8966, -68.5908) -> (-19.9215, -68.6136) construction
  spline S51 degree 5 poles (-56.0345, 24.1948) (-56.0628, 24.2071) (-56.1198, 24.2308) (-56.2062, 24.264) (-56.3229, 24.3039) (-56.4711, 24.3478) (-56.6208, 24.3873) (-56.7714, 24.4241) (-56.9226, 24.4595) (-57.0741, 24.494) (-57.226, 24.5274) (-57.3783, 24.5594) (-57.5312, 24.5896) (-57.6848, 24.6176) (-57.8391, 24.6435) (-57.994, 24.6674) (-58.1494, 24.6897) (-58.3052, 24.7105) (-58.4614, 24.7301) (-58.6179, 24.7485) (-58.7747, 24.7658) (-58.9318, 24.7818) (-59.0893, 24.7965) (-59.2471, 24.8098) (-59.4053, 24.8218) (-59.5638, 24.8325) (-59.7226, 24.842) (-59.8817, 24.8504) (-60.0411, 24.8577) (-60.2007, 24.8638) (-60.3605, 24.8689) (-60.5206, 24.8729) (-60.6809, 24.8757) (-60.8415, 24.8776) (-61.0023, 24.8783) (-61.1633, 24.878) (-61.3245, 24.8766) (-61.4859, 24.8742) (-61.6475, 24.8708) (-61.8093, 24.8665) (-61.9712, 24.8611) (-62.1334, 24.8548) (-62.2957, 24.8475) (-62.4581, 24.8392) (-62.6207, 24.83) (-62.7835, 24.8199) (-62.9464, 24.8088) (-63.1095, 24.7967) (-63.2727, 24.7838) (-63.436, 24.77) (-63.5995, 24.7552) (-63.7631, 24.7396) (-63.9268, 24.723) (-64.0906, 24.7056) (-64.2545, 24.6873) (-64.4185, 24.6681) (-64.5826, 24.648) (-64.7468, 24.6271) (-64.9111, 24.6054) (-65.0755, 24.5828) (-65.24, 24.5593) (-65.4046, 24.535) (-65.5692, 24.5098) (-65.734, 24.4839) (-65.8987, 24.4571) (-66.0636, 24.4294) (-66.2285, 24.401) (-66.3935, 24.3718) (-66.5585, 24.3417) (-66.7236, 24.3108) (-66.8887, 24.2792) (-67.0208, 24.2532) (-67.1199, 24.2334) (-67.186, 24.22) (-67.2191, 24.2132) knots 0 0 0 0 0 0 0.01428571 0.02857143 0.04285714 0.05714286 0.07142857 0.08571429 0.1 0.11428571 0.12857143 0.14285714 0.15714286 0.17142857 0.18571429 0.2 0.21428571 0.22857143 0.24285714 0.25714286 0.27142857 0.28571429 0.3 0.31428571 0.32857143 0.34285714 0.35714286 0.37142857 0.38571429 0.4 0.41428571 0.42857143 0.44285714 0.45714286 0.47142857 0.48571429 0.5 0.51428571 0.52857143 0.54285714 0.55714286 0.57142857 0.58571429 0.6 0.61428571 0.62857143 0.64285714 0.65714286 0.67142857 0.68571429 0.7 0.71428571 0.72857143 0.74285714 0.75714286 0.77142857 0.78571429 0.8 0.81428571 0.82857143 0.84285714 0.85714286 0.87142857 0.88571429 0.9 0.91428571 0.92857143 0.94285714 0.95714286 0.97142857 0.98571429 1 1 1 1 1 1
  line L3820 (-56.0345, 24.1948) -> (-56.0628, 24.2071) construction
  line L3821 (-56.0628, 24.2071) -> (-56.1198, 24.2308) construction
  line L3822 (-56.1198, 24.2308) -> (-56.2062, 24.264) construction
  line L3823 (-56.2062, 24.264) -> (-56.3229, 24.3039) construction
  line L3824 (-56.3229, 24.3039) -> (-56.4711, 24.3478) construction
  line L3825 (-56.4711, 24.3478) -> (-56.6208, 24.3873) construction
  line L3826 (-56.6208, 24.3873) -> (-56.7714, 24.4241) construction
  line L3827 (-56.7714, 24.4241) -> (-56.9226, 24.4595) construction
  line L3828 (-56.9226, 24.4595) -> (-57.0741, 24.494) construction
  line L3829 (-57.0741, 24.494) -> (-57.226, 24.5274) construction
  line L3830 (-57.226, 24.5274) -> (-57.3783, 24.5594) construction
  line L3831 (-57.3783, 24.5594) -> (-57.5312, 24.5896) construction
  line L3832 (-57.5312, 24.5896) -> (-57.6848, 24.6176) construction
  line L3833 (-57.6848, 24.6176) -> (-57.8391, 24.6435) construction
  line L3834 (-57.8391, 24.6435) -> (-57.994, 24.6674) construction
  line L3835 (-57.994, 24.6674) -> (-58.1494, 24.6897) construction
  line L3836 (-58.1494, 24.6897) -> (-58.3052, 24.7105) construction
  line L3837 (-58.3052, 24.7105) -> (-58.4614, 24.7301) construction
  line L3838 (-58.4614, 24.7301) -> (-58.6179, 24.7485) construction
  line L3839 (-58.6179, 24.7485) -> (-58.7747, 24.7658) construction
  line L3840 (-58.7747, 24.7658) -> (-58.9318, 24.7818) construction
  line L3841 (-58.9318, 24.7818) -> (-59.0893, 24.7965) construction
  line L3842 (-59.0893, 24.7965) -> (-59.2471, 24.8098) construction
  line L3843 (-59.2471, 24.8098) -> (-59.4053, 24.8218) construction
  line L3844 (-59.4053, 24.8218) -> (-59.5638, 24.8325) construction
  line L3845 (-59.5638, 24.8325) -> (-59.7226, 24.842) construction
  line L3846 (-59.7226, 24.842) -> (-59.8817, 24.8504) construction
  line L3847 (-59.8817, 24.8504) -> (-60.0411, 24.8577) construction
  line L3848 (-60.0411, 24.8577) -> (-60.2007, 24.8638) construction
  line L3849 (-60.2007, 24.8638) -> (-60.3605, 24.8689) construction
  line L3850 (-60.3605, 24.8689) -> (-60.5206, 24.8729) construction
  line L3851 (-60.5206, 24.8729) -> (-60.6809, 24.8757) construction
  line L3852 (-60.6809, 24.8757) -> (-60.8415, 24.8776) construction
  line L3853 (-60.8415, 24.8776) -> (-61.0023, 24.8783) construction
  line L3854 (-61.0023, 24.8783) -> (-61.1633, 24.878) construction
  line L3855 (-61.1633, 24.878) -> (-61.3245, 24.8766) construction
  line L3856 (-61.3245, 24.8766) -> (-61.4859, 24.8742) construction
  line L3857 (-61.4859, 24.8742) -> (-61.6475, 24.8708) construction
  line L3858 (-61.6475, 24.8708) -> (-61.8093, 24.8665) construction
  line L3859 (-61.8093, 24.8665) -> (-61.9712, 24.8611) construction
  line L3860 (-61.9712, 24.8611) -> (-62.1334, 24.8548) construction
  line L3861 (-62.1334, 24.8548) -> (-62.2957, 24.8475) construction
  line L3862 (-62.2957, 24.8475) -> (-62.4581, 24.8392) construction
  line L3863 (-62.4581, 24.8392) -> (-62.6207, 24.83) construction
  line L3864 (-62.6207, 24.83) -> (-62.7835, 24.8199) construction
  line L3865 (-62.7835, 24.8199) -> (-62.9464, 24.8088) construction
  line L3866 (-62.9464, 24.8088) -> (-63.1095, 24.7967) construction
  line L3867 (-63.1095, 24.7967) -> (-63.2727, 24.7838) construction
  line L3868 (-63.2727, 24.7838) -> (-63.436, 24.77) construction
  line L3869 (-63.436, 24.77) -> (-63.5995, 24.7552) construction
  line L3870 (-63.5995, 24.7552) -> (-63.7631, 24.7396) construction
  line L3871 (-63.7631, 24.7396) -> (-63.9268, 24.723) construction
  line L3872 (-63.9268, 24.723) -> (-64.0906, 24.7056) construction
  line L3873 (-64.0906, 24.7056) -> (-64.2545, 24.6873) construction
  line L3874 (-64.2545, 24.6873) -> (-64.4185, 24.6681) construction
  line L3875 (-64.4185, 24.6681) -> (-64.5826, 24.648) construction
  line L3876 (-64.5826, 24.648) -> (-64.7468, 24.6271) construction
  line L3877 (-64.7468, 24.6271) -> (-64.9111, 24.6054) construction
  line L3878 (-64.9111, 24.6054) -> (-65.0755, 24.5828) construction
  line L3879 (-65.0755, 24.5828) -> (-65.24, 24.5593) construction
  line L3880 (-65.24, 24.5593) -> (-65.4046, 24.535) construction
  line L3881 (-65.4046, 24.535) -> (-65.5692, 24.5098) construction
  line L3882 (-65.5692, 24.5098) -> (-65.734, 24.4839) construction
  line L3883 (-65.734, 24.4839) -> (-65.8987, 24.4571) construction
  line L3884 (-65.8987, 24.4571) -> (-66.0636, 24.4294) construction
  line L3885 (-66.0636, 24.4294) -> (-66.2285, 24.401) construction
  line L3886 (-66.2285, 24.401) -> (-66.3935, 24.3718) construction
  line L3887 (-66.3935, 24.3718) -> (-66.5585, 24.3417) construction
  line L3888 (-66.5585, 24.3417) -> (-66.7236, 24.3108) construction
  line L3889 (-66.7236, 24.3108) -> (-66.8887, 24.2792) construction
  line L3890 (-66.8887, 24.2792) -> (-67.0208, 24.2532) construction
  line L3891 (-67.0208, 24.2532) -> (-67.1199, 24.2334) construction
  line L3892 (-67.1199, 24.2334) -> (-67.186, 24.22) construction
  line L3893 (-67.186, 24.22) -> (-67.2191, 24.2132) construction
  arc A93 (43.8, 56.4469) -> (40.1492, 59.0993) centre (0, 0) ccw
  arc A94 (71.4115, -2.2563) -> (71.4115, 2.2563) centre (0, 0) ccw
  arc A95 (24.5301, -51.9354) -> (27.5982, -50.3721) centre (0, 0) ccw
  arc A96 (10.6816, 56.435) -> (7.2806, 56.9737) centre (0, 0) ccw
  arc A97 (-7.2806, 56.9737) -> (-10.6816, 56.435) centre (0, 0) ccw
  line L3894 (-13.005, -57.9623) -> (-13.3622, -59.5542)
  line L3895 (-51.1066, -30.2798) -> (-52.5103, -31.1115)
  line L3896 (-59.1442, -5.5428) -> (-60.7685, -5.6951)
  spline S52 degree 5 poles (59.5542, -13.3622) (59.5843, -13.369) (59.6444, -13.3833) (59.7338, -13.4071) (59.8517, -13.4435) (59.9973, -13.4951) (60.1416, -13.5511) (60.2852, -13.6099) (60.4283, -13.6701) (60.5711, -13.7313) (60.7136, -13.7935) (60.8557, -13.8571) (60.9971, -13.9226) (61.1379, -13.9902) (61.2779, -14.06) (61.4173, -14.1316) (61.5561, -14.205) (61.6944, -14.2797) (61.8322, -14.3557) (61.9697, -14.4327) (62.1067, -14.5109) (62.2432, -14.5904) (62.3792, -14.6711) (62.5148, -14.753) (62.6498, -14.8363) (62.7843, -14.9208) (62.9184, -15.0064) (63.052, -15.0932) (63.1852, -15.181) (63.318, -15.2698) (63.4503, -15.3597) (63.5821, -15.4506) (63.7135, -15.5425) (63.8445, -15.6354) (63.975, -15.7293) (64.105, -15.8242) (64.2346, -15.92) (64.3638, -16.0168) (64.4926, -16.1146) (64.6209, -16.2132) (64.7488, -16.3127) (64.8762, -16.4131) (65.0032, -16.5144) (65.1298, -16.6166) (65.256, -16.7196) (65.3817, -16.8235) (65.507, -16.9283) (65.6318, -17.0338) (65.7562, -17.1402) (65.8802, -17.2474) (66.0038, -17.3555) (66.1269, -17.4643) (66.2497, -17.5739) (66.3719, -17.6842) (66.4938, -17.7954) (66.6152, -17.9073) (66.7362, -18.02) (66.8568, -18.1335) (66.9769, -18.2477) (67.0966, -18.3626) (67.2159, -18.4782) (67.3347, -18.5946) (67.4531, -18.7118) (67.5711, -18.8296) (67.6887, -18.9481) (67.8058, -19.0674) (67.9225, -19.1873) (68.0388, -19.3079) (68.1546, -19.4293) (68.27, -19.5512) (68.385, -19.6739) (68.4767, -19.7726) (68.5452, -19.8469) (68.5908, -19.8966) (68.6136, -19.9215) knots 0 0 0 0 0 0 0.01428571 0.02857143 0.04285714 0.05714286 0.07142857 0.08571429 0.1 0.11428571 0.12857143 0.14285714 0.15714286 0.17142857 0.18571429 0.2 0.21428571 0.22857143 0.24285714 0.25714286 0.27142857 0.28571429 0.3 0.31428571 0.32857143 0.34285714 0.35714286 0.37142857 0.38571429 0.4 0.41428571 0.42857143 0.44285714 0.45714286 0.47142857 0.48571429 0.5 0.51428571 0.52857143 0.54285714 0.55714286 0.57142857 0.58571429 0.6 0.61428571 0.62857143 0.64285714 0.65714286 0.67142857 0.68571429 0.7 0.71428571 0.72857143 0.74285714 0.75714286 0.77142857 0.78571429 0.8 0.81428571 0.82857143 0.84285714 0.85714286 0.87142857 0.88571429 0.9 0.91428571 0.92857143 0.94285714 0.95714286 0.97142857 0.98571429 1 1 1 1 1 1
  line L3897 (59.5542, -13.3622) -> (59.5843, -13.369) construction
  line L3898 (59.5843, -13.369) -> (59.6444, -13.3833) construction
  line L3899 (59.6444, -13.3833) -> (59.7338, -13.4071) construction
  line L3900 (59.7338, -13.4071) -> (59.8517, -13.4435) construction
  line L3901 (59.8517, -13.4435) -> (59.9973, -13.4951) construction
  line L3902 (59.9973, -13.4951) -> (60.1416, -13.5511) construction
  line L3903 (60.1416, -13.5511) -> (60.2852, -13.6099) construction
  line L3904 (60.2852, -13.6099) -> (60.4283, -13.6701) construction
  line L3905 (60.4283, -13.6701) -> (60.5711, -13.7313) construction
  line L3906 (60.5711, -13.7313) -> (60.7136, -13.7935) construction
  line L3907 (60.7136, -13.7935) -> (60.8557, -13.8571) construction
  line L3908 (60.8557, -13.8571) -> (60.9971, -13.9226) construction
  line L3909 (60.9971, -13.9226) -> (61.1379, -13.9902) construction
  line L3910 (61.1379, -13.9902) -> (61.2779, -14.06) construction
  line L3911 (61.2779, -14.06) -> (61.4173, -14.1316) construction
  line L3912 (61.4173, -14.1316) -> (61.5561, -14.205) construction
  line L3913 (61.5561, -14.205) -> (61.6944, -14.2797) construction
  line L3914 (61.6944, -14.2797) -> (61.8322, -14.3557) construction
  line L3915 (61.8322, -14.3557) -> (61.9697, -14.4327) construction
  line L3916 (61.9697, -14.4327) -> (62.1067, -14.5109) construction
  line L3917 (62.1067, -14.5109) -> (62.2432, -14.5904) construction
  line L3918 (62.2432, -14.5904) -> (62.3792, -14.6711) construction
  line L3919 (62.3792, -14.6711) -> (62.5148, -14.753) construction
  line L3920 (62.5148, -14.753) -> (62.6498, -14.8363) construction
  line L3921 (62.6498, -14.8363) -> (62.7843, -14.9208) construction
  line L3922 (62.7843, -14.9208) -> (62.9184, -15.0064) construction
  line L3923 (62.9184, -15.0064) -> (63.052, -15.0932) construction
  line L3924 (63.052, -15.0932) -> (63.1852, -15.181) construction
  line L3925 (63.1852, -15.181) -> (63.318, -15.2698) construction
  line L3926 (63.318, -15.2698) -> (63.4503, -15.3597) construction
  line L3927 (63.4503, -15.3597) -> (63.5821, -15.4506) construction
  line L3928 (63.5821, -15.4506) -> (63.7135, -15.5425) construction
  line L3929 (63.7135, -15.5425) -> (63.8445, -15.6354) construction
  line L3930 (63.8445, -15.6354) -> (63.975, -15.7293) construction
  line L3931 (63.975, -15.7293) -> (64.105, -15.8242) construction
  line L3932 (64.105, -15.8242) -> (64.2346, -15.92) construction
  line L3933 (64.2346, -15.92) -> (64.3638, -16.0168) construction
  line L3934 (64.3638, -16.0168) -> (64.4926, -16.1146) construction
  line L3935 (64.4926, -16.1146) -> (64.6209, -16.2132) construction
  line L3936 (64.6209, -16.2132) -> (64.7488, -16.3127) construction
  line L3937 (64.7488, -16.3127) -> (64.8762, -16.4131) construction
  line L3938 (64.8762, -16.4131) -> (65.0032, -16.5144) construction
  line L3939 (65.0032, -16.5144) -> (65.1298, -16.6166) construction
  line L3940 (65.1298, -16.6166) -> (65.256, -16.7196) construction
  line L3941 (65.256, -16.7196) -> (65.3817, -16.8235) construction
  line L3942 (65.3817, -16.8235) -> (65.507, -16.9283) construction
  line L3943 (65.507, -16.9283) -> (65.6318, -17.0338) construction
  line L3944 (65.6318, -17.0338) -> (65.7562, -17.1402) construction
  line L3945 (65.7562, -17.1402) -> (65.8802, -17.2474) construction
  line L3946 (65.8802, -17.2474) -> (66.0038, -17.3555) construction
  line L3947 (66.0038, -17.3555) -> (66.1269, -17.4643) construction
  line L3948 (66.1269, -17.4643) -> (66.2497, -17.5739) construction
  line L3949 (66.2497, -17.5739) -> (66.3719, -17.6842) construction
  line L3950 (66.3719, -17.6842) -> (66.4938, -17.7954) construction
  line L3951 (66.4938, -17.7954) -> (66.6152, -17.9073) construction
  line L3952 (66.6152, -17.9073) -> (66.7362, -18.02) construction
  line L3953 (66.7362, -18.02) -> (66.8568, -18.1335) construction
  line L3954 (66.8568, -18.1335) -> (66.9769, -18.2477) construction
  line L3955 (66.9769, -18.2477) -> (67.0966, -18.3626) construction
  line L3956 (67.0966, -18.3626) -> (67.2159, -18.4782) construction
  line L3957 (67.2159, -18.4782) -> (67.3347, -18.5946) construction
  line L3958 (67.3347, -18.5946) -> (67.4531, -18.7118) construction
  line L3959 (67.4531, -18.7118) -> (67.5711, -18.8296) construction
  line L3960 (67.5711, -18.8296) -> (67.6887, -18.9481) construction
  line L3961 (67.6887, -18.9481) -> (67.8058, -19.0674) construction
  line L3962 (67.8058, -19.0674) -> (67.9225, -19.1873) construction
  line L3963 (67.9225, -19.1873) -> (68.0388, -19.3079) construction
  line L3964 (68.0388, -19.3079) -> (68.1546, -19.4293) construction
  line L3965 (68.1546, -19.4293) -> (68.27, -19.5512) construction
  line L3966 (68.27, -19.5512) -> (68.385, -19.6739) construction
  line L3967 (68.385, -19.6739) -> (68.4767, -19.7726) construction
  line L3968 (68.4767, -19.7726) -> (68.5452, -19.8469) construction